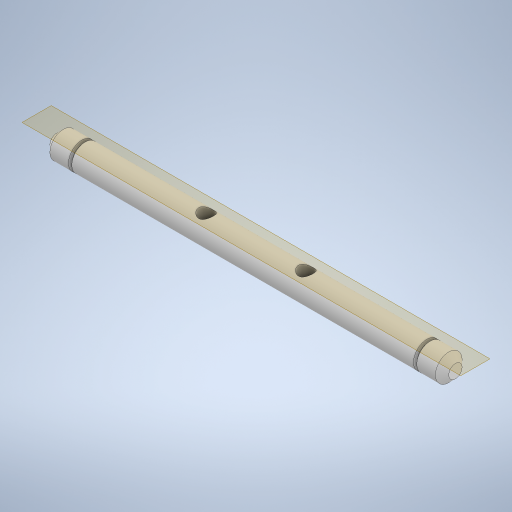
# Autodesk Inventor part: axle
Saved by Autodesk Inventor 2023 (Build 270158000, 158)
## iProperties
Created: 2023-10-25
Part Number: axle
Material: Generic
Document SubType Name: Modeling
Designer: mirek
Density: 1 g/cm^3
Appearance: Default
Author: mirek
Autodesk Inventor part; units mm, degrees
ref_plane "YZ Plane" through (0, 0, 0) normal (1, 0, 0) x (0, 1, 0)
ref_plane "XY Plane" through (0, 0, 0) normal (0, 0, 1) x (1, 0, 0)
sketch "Sketch2" plane through (0, 0, 0) normal (0, 0, 1) x (1, 0, 0)
  line L0 (-15, 1) -> (-15, 0)
  line L1 (-15, 0) -> (15, 0)
  line L2 (15, 0) -> (15, 1)
  line L3 (15, 1) -> (-15, 1)
  line L4 (-15, 1) -> (15, 0) construction
  line L5 (-15, 0) -> (15, 1) construction
  line L6 (-13.1, 1) -> (-12.85, 1)
  line L7 (-12.85, 1) -> (-12.85, 0.7)
  line L8 (-12.85, 0.7) -> (-13.1, 0.7)
  line L9 (-13.1, 0.7) -> (-13.1, 1)
  line L10 (0, 0) -> (0, 1)
  line L11 (12.85, 1) -> (12.85, 0.7)
  line L12 (12.85, 0.7) -> (13.1, 0.7)
  line L13 (13.1, 0.7) -> (13.1, 1)
  line L14 (-21, 0) -> (21, 0) projected
  point P0 (0, 0.5)
  point P1 (0, 0.5)
  dimension "d1" = 1
  dimension "d2" = 30
  dimension "d3" = 0.25
  dimension "d4" = 0.3
  dimension "d5" = 25.7
  constraints: 28 end point, 5 midpoint, 4 parallel, 4 symmetric about line, 2 perpendicular, 1 horizontal, 1 point on line, 1 vertical, 1 vertical alignment
  measures "d1" distance of L1.end L2.end
  measures "d2" distance of L2.end L0.start
  measures "d3" distance of L7.end L8.end
  measures "d4" distance of L8.end L6.start
  measures "d5" distance between parallel lines of L11 L7
revolve "Revolution1" add sketch "Sketch2" angle 360 about axis through (-10, 0, 0) along (1, 0, 0) contours L3 L9 L8 L7 L10 L1 L0 | L10 L3 L11 L12 L13 L2 L1
ref_plane "Work Plane1" through (0, 1, 0) normal (0, 1, 0) x (-1, 0, 0)
sketch "Sketch3" plane through (0, 1, 0) normal (0, 1, 0) x (-1, 0, 0)
  circle A0 centre (3.75, 0) radius 0.55
  line L0 (0, 0.9388) -> (0, -0.9388)
  circle A1 centre (-3.75, 0) radius 0.55
  point P0 (0, 0)
  point P1 (0, 0)
  dimension "d10" = 1.1
  dimension "d11" = 7.5
  constraints: 2 centre point, 2 end point, 1 coincident, 1 horizontal alignment, 1 midpoint, 1 symmetric about line, 1 vertical, 1 other
  measures "d10" diameter of A0
  measures "d11" distance of A1.centre A0.centre
extrude "Extrusion1" cut sketch "Sketch3" against normal through all
chamfer "Chamfer1" distance 0.5 angle 45 2 edges at (-15, -1, 0) (15, -1, 0)
body "Solid1"
